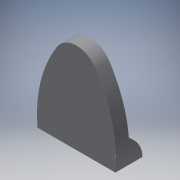
# Autodesk Inventor part: HeadFrame
Saved by Autodesk Inventor 2016 (Build 200138000, 138)
## iProperties
Created: 2017-03-13
Part Number: HeadFrame
Material: Generic
Document SubType Name: Modeling
Designer: Owner
Density: 1 g/cm^3
Appearance: Default
Author: Owner
Autodesk Inventor part; units mm, degrees
ref_plane "YZ Plane" through (0, 0, 0) normal (1, 0, 0) x (0, 1, 0)
ref_plane "XZ Plane" through (0, 0, 0) normal (0, 1, 0) x (-1, 0, 0)
ref_plane "XY Plane" through (0, 0, 0) normal (0, 0, 1) x (1, 0, 0)
sketch "Sketch1" plane through (0, 0, 0) normal (0, 0, 1) x (1, 0, 0)
  line L0 (43.1, 62.15) -> (-43.1, 62.15) projected
  line L1 (43.1, 62.15) -> (-43.1, 62.15)
  line L2 (-43.1, 62.15) -> (-43.1, 176.45)
  line L3 (-43.1, 176.45) -> (43.1, 176.45)
  line L4 (43.1, 176.45) -> (43.1, 62.15)
  arc A0 (43.1, 62.15) -> (21.3882, 150.6616) centre (-96.2036, 74.8977) ccw
  arc A1 (-21.3307, 150.6382) -> (-43.1, 62.15) centre (96.939, 74.6204) ccw
  arc A2 (21.3882, 150.6616) -> (-21.3307, 150.6382) centre (0.0363, 136.9046) ccw
  point P0 (0, 0)
  dimension "d0" = 114.3
  dimension "d1" = 25.4
  constraints: 8 end point, 6 point on circle, 3 centre point, 2 parallel, 2 tangent, 1 horizontal, 1 perpendicular
  measures "d0" distance of L3.end L0.start
  measures "d1" radius of A2
extrude "Extrusion1" add sketch "Sketch1" against normal blind 5 contours L0 L2 A1 A2 A0 L4 | L4 A0 | A1 L2
sketch "Sketch2" plane through (0, 0, -5) normal (0, 0, -1) x (-1, 0, 0)
  arc A0 (-21.3882, 150.6616) -> (-43.1, 62.15) centre (96.2036, 74.8977) ccw projected
  line L0 (-43.1, 62.15) -> (43.1, 62.15) projected
  arc A1 (43.1, 62.15) -> (21.3307, 150.6382) centre (-96.939, 74.6204) ccw projected
  arc A2 (21.3307, 150.6382) -> (-21.3882, 150.6616) centre (-0.0363, 136.9046) ccw projected
  arc A3 (-16.0502, 147.2223) -> (-32.7704, 90.1915) centre (72.1437, 90.3994) ccw
  arc A4 (32.7315, 90.1915) -> (15.989, 147.2048) centre (-72.7133, 90.1915) ccw
  arc A5 (15.989, 147.2048) -> (-16.0502, 147.2223) centre (-0.0363, 136.9046) ccw
  line L1 (-43.1, 62.15) -> (43.1, 62.15) projected
  line L2 (-32.3341, 62.15) -> (32.3159, 62.15)
  line L3 (32.7315, 90.1915) -> (32.7315, 62.15)
  line L4 (32.7315, 62.15) -> (-32.7704, 62.15)
  line L5 (-32.7704, 62.15) -> (-32.7704, 90.1915)
  point P0 (0, 0)
  constraints: 8 end point, 6 point on circle, 3 centre point, 2 point on line, 1 parallel
extrude "Extrusion2" add sketch "Sketch2" along normal blind 10 contours A2 A1 L0 L3 A4 A5 A3 L5 A0
sketch "Sketch3" plane through (-32.7315, 62.15, -5) normal (1, 0, 0) x (0, 0, -1)
  line L0 (0, 0) -> (25, 0)
  line L1 (-5, 0) -> (10, 0) projected
  line L2 (10, 0) -> (10, 25.4)
  arc A0 (25, 0) -> (10, 25.4) centre (-9.2015, -3.0686) ccw
  line L3 (10, 25.4) -> (10, -0.6619)
  line L4 (25, 0) -> (10, 0)
  line L5 (10, 0) -> (10, 25.4)
  point P0 (-5, -62.15)
  dimension "d6" = 25
  dimension "d7" = 25.4
  constraints: 10 end point, 2 collinear, 2 perpendicular, 2 point on circle, 1 centre point, 1 vertical
  measures "d6" distance of L0.start L0.end
  measures "d7" distance of L1.end L2.end
extrude "Extrusion3" add sketch "Sketch3" along normal blind 101.6 and the other way blind 25.4
sketch "Sketch4" plane through (0, 0, -15) normal (0, 0, -1) x (-1, 0, 0)
  line L0 (32.7315, 62.15) -> (32.7315, 90.1915) projected
  arc A0 (32.7315, 90.1915) -> (15.989, 147.2048) centre (-72.7133, 90.1915) ccw projected
  arc A1 (15.989, 147.2048) -> (-16.0502, 147.2223) centre (-0.0363, 136.9046) ccw projected
  arc A2 (-16.0502, 147.2223) -> (-32.7704, 90.1915) centre (72.1437, 90.3994) ccw projected
  line L1 (-32.7704, 90.1915) -> (-32.7704, 62.15) projected
  line L2 (-32.7704, 62.15) -> (32.7315, 62.15) projected
  arc A3 (-21.3882, 150.6616) -> (-43.1087, 87.55) centre (96.2036, 74.8977) ccw projected
  line L3 (-21.3882, 150.6616) -> (-130.3093, 136.9046)
  line L4 (-130.3093, 136.9046) -> (-112.871, 20.9919)
  arc A4 (-21.3882, 150.6616) -> (-43.1, 62.15) centre (96.2036, 74.8977) ccw projected
  line L5 (-43.1, 62.15) -> (-112.871, 20.9919)
  arc A5 (43.0584, 87.55) -> (21.3307, 150.6382) centre (-96.939, 74.6204) ccw projected
  line L6 (21.3307, 150.6382) -> (115.9935, 147.2223)
  line L7 (115.9935, 147.2223) -> (119.9418, 13.6964)
  line L8 (119.9418, 13.6964) -> (43.1, 62.15)
  arc A6 (43.1, 62.15) -> (43.0584, 87.55) centre (-96.939, 74.6204) ccw projected
  point P0 (0, 0)
  constraints: 12 end point, 1 point on circle
extrude "Extrusion4" cut sketch "Sketch4" along normal blind 25.4
sketch "Sketch5" plane through (0, 0, -15) normal (0, 0, -1) x (-1, 0, 0)
  arc A0 (15.989, 147.2048) -> (-16.0502, 147.2223) centre (-0.0363, 136.9046) ccw projected
  line L0 (32.7315, 62.15) -> (32.7315, 90.1915) projected
  arc A1 (32.7315, 90.1915) -> (15.989, 147.2048) centre (-72.7133, 90.1915) ccw projected
  arc A2 (15.989, 147.2048) -> (-16.0502, 147.2223) centre (-0.0363, 136.9046) ccw projected
  arc A3 (-16.0502, 147.2223) -> (-32.7704, 90.1915) centre (72.1437, 90.3994) ccw projected
  line L1 (-32.7704, 90.1915) -> (-32.7704, 62.15) projected
  line L2 (-32.7704, 62.15) -> (32.7315, 62.15) projected
  arc A4 (43.0584, 87.55) -> (21.3307, 150.6382) centre (-96.939, 74.6204) ccw projected
  arc A5 (21.3307, 150.6382) -> (-21.3882, 150.6616) centre (-0.0363, 136.9046) ccw projected
  arc A6 (-21.3882, 150.6616) -> (-43.1087, 87.55) centre (96.2036, 74.8977) ccw projected
  line L3 (-0.0259, 155.9546) -> (11.9455, 151.7147)
  line L4 (-0.0259, 155.9546) -> (2.1885, 162.207)
  line L5 (11.9455, 151.7147) -> (14.1599, 157.9671)
  line L6 (14.1599, 157.9671) -> (2.1885, 162.207)
  line L7 (11.9455, 151.7147) -> (19.4303, 141.4571)
  arc A7 (32.7315, 90.1915) -> (15.989, 147.2048) centre (-72.7133, 90.1915) ccw projected
  line L8 (11.9455, 151.7147) -> (17.2075, 155.5543)
  line L9 (19.4303, 141.4571) -> (24.6263, 145.2485)
  line L10 (17.2075, 155.5543) -> (24.6263, 145.2485)
  point P0 (0, 0)
  dimension "d14" = 12.7
  constraints: 16 end point, 9 point on circle, 2 perpendicular
  measures "d14" distance of L3.start L3.end
body "Solid1"
